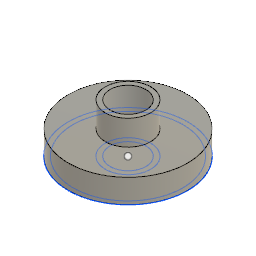
PixelFace v3 (Autodesk Fusion 360 design; units mm, degrees)
Autodesk Fusion 360 part; units mm, degrees
sketch "Sketch1" plane through (0, 0, 0) normal (0, 0, 1) x (1, 0, 0) in component "base"
  circle A0 centre (43.9809, 31.3929) radius 50
  circle A1 centre (43.9809, 31.3929) radius 46
  circle A2 centre (43.9809, 31.3929) radius 19
  circle A3 centre (43.9809, 31.3929) radius 15
  dimension "d1" = 100
  dimension "d2" = 4
  dimension "d4" = 4
  dimension "d6" = 30
  measures "d1" diameter of A0
  measures "d2" distance of A0 A1
  measures "d4" distance of A2 A3
  measures "d6" diameter of A3
extrude "Extrude1" add sketch "Sketch1" against normal blind 20 contours A0 | A1 makes body 1 in component "base"
extrude "Extrude2" cut sketch "Sketch1" against normal blind 16 contours A1 bodies 1 in component "base"
extrude "Extrude3" add sketch "Sketch1" against normal blind 25 from surface at -16 contours A2 bodies 1 in component "base"
move_body "Move1" bodies 1 to x (1, 0, 0) y (0, -1, 0) z (0, 0, -1) at (0, -37.2143, -80) in component "base"
move_body "Move2" bodies 1 to x (1, 0, 0) y (0, 1, 0) z (0, 0, 1) at (0, 100, 80) in component "base"
copy_body "CutPasteBodies1" bodies 1 removing the originals makes body 2 in component "base"
component "base" placed x (1, 0, 0) y (0, 1, 0) z (0, 0, 1) at (0, 0, 0)
component "Component" placed x (1, 0, 0) y (0, 1, 0) z (0, 0, 1) at (0, 0, 0)
equation "d2 = wallthickness"
equation "wallthickness = 4 mm"
equation "d4 = wallthickness"
equation "motorDiameter = 30 mm"
equation "d6 = motorDiameter"
equation "baseHeight = 20 mm"
equation "motorBaseHeight = 25 mm"
equation "d9 = -baseHeight"
equation "d11 = wallthickness - baseHeight"
equation "d13 = -baseHeight + wallthickness"
equation "d14 = -motorBaseHeight"
